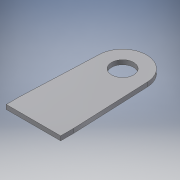
# Autodesk Inventor part: 足裏_メインフレーム_1_1
Saved by Autodesk Inventor 2018 (Build 220112000, 112)
## iProperties
Created: 2016-05-01
Part Number: 足裏_メインフレーム_1_1
Material: アルミニウム 2014-T4
Document SubType Name: Modeling
Designer: hiroaki
Density: 2.8 g/cm^3
Appearance: サテン
Mass: 5.80863 g
Surface Area: 25.475 cm^2
Volume: 2.07451 cm^3
Author: hiroaki
Autodesk Inventor part; units mm, degrees
ref_plane "YZ Plane" through (0, 0, 0) normal (1, 0, 0) x (0, 1, 0)
ref_plane "XZ Plane" through (0, 0, 0) normal (0, 1, 0) x (-1, 0, 0)
ref_plane "XY Plane" through (0, 0, 0) normal (0, 0, 1) x (1, 0, 0)
derived "足裏_基礎_1.ipt"
sketch "スケッチ1" plane through (0, 0, 0) normal (0, 0, 1) x (1, 0, 0)
  circle A0 centre (0, 0) radius 5.05
  line L0 (-21.25, 26.6) -> (21.25, 26.6) construction
  line L1 (21.25, 26.6) -> (21.25, -16) construction
  line L2 (21.25, -16) -> (-21.25, -16) construction
  line L3 (-21.25, -16) -> (-21.25, 26.6) construction
  circle A1 centre (0, 0) radius 26.6 construction
  line L4 (-12.5, -41) -> (12.5, -41)
  line L5 (12.5, -41) -> (12.5, -35)
  line L6 (12.5, -35) -> (10.99, 0.4679)
  line L7 (-12.5, -41) -> (-12.5, -35)
  line L8 (-12.5, -35) -> (-10.99, 0.4679)
  arc A2 (10.99, 0.4679) -> (-10.99, 0.4679) centre (0, 0) ccw
  line L9 (12.5, -35) -> (-12.5, -35) construction
  circle A3 centre (0, 8.5) radius 1.35
  circle A4 centre (0, 8.5) radius 2.5 construction
  circle A5 centre (-8.5, 0) radius 1.35
  circle A6 centre (0, -8.5) radius 1.35
  circle A7 centre (8.5, 0) radius 1.35
  circle A8 centre (-9.5, -38) radius 1.55
  circle A9 centre (0, -38) radius 1.55
  circle A10 centre (9.5, -38) radius 1.55
  line L10 (-12.5, -38) -> (12.5, -38) construction
  line L11 (0, 0) -> (0, -35) construction
  line L12 (-6.3, -35) -> (-3.2, -35) construction
  line L13 (-3.2, -35) -> (-3.2, -41) construction
  line L14 (-3.2, -41) -> (-6.3, -41) construction
  line L15 (-6.3, -41) -> (-6.3, -35) construction
  line L16 (3.2, -35) -> (6.3, -35) construction
  line L17 (6.3, -35) -> (6.3, -41) construction
  line L18 (6.3, -41) -> (3.2, -41) construction
  line L19 (3.2, -41) -> (3.2, -35) construction
  line L20 (-4.75, -35) -> (-4.75, -41) construction
  line L21 (4.75, -35) -> (4.75, -41) construction
  point P0 (0, 26.6)
  point P1 (0, -41)
extrude "押し出し1" add sketch "スケッチ1" along normal blind 2
sketch "スケッチ3" plane through (0, 0, 0) normal (0, 0, -1) x (-1, 0, 0)
  circle A0 centre (0, -8.5) radius 1.35 projected
  circle A1 centre (0, -8.5) radius 1.35
  circle A2 centre (8.5, 0) radius 1.35 projected
  circle A3 centre (8.5, 0) radius 1.35
  circle A4 centre (-8.5, 0) radius 1.35 projected
  circle A5 centre (-8.5, 0) radius 1.35
  circle A6 centre (0, 8.5) radius 1.35 projected
  circle A7 centre (0, 8.5) radius 1.35
  circle A8 centre (0, -38) radius 1.55 projected
  circle A9 centre (0, -38) radius 1.55
  circle A10 centre (-9.5, -38) radius 1.55 projected
  circle A11 centre (-9.5, -38) radius 1.55
  circle A12 centre (9.5, -38) radius 1.55 projected
  circle A13 centre (9.5, -38) radius 1.55
  point P0 (0, 0)
  constraints: 7 centre point, 7 coincident
extrude "押し出し2" add sketch "スケッチ3" against normal up to surface (2 mm away)
